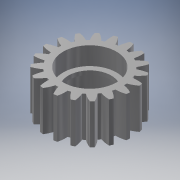
# Autodesk Inventor part: planet2_2
Saved by Autodesk Inventor 2019 (Build 230136000, 136)
## iProperties
Created: 2019-12-31
Part Number: planet2_2
Material: Steel
Document SubType Name: Modeling
Designer: louis
Categories: <?xml version="1.0" encoding="UTF-16"?> <MemberInstance><Categories><FamilyTemplate><FamilyTemplateParameter ValueType="xs:double" Id="1" ObjectReferenceKey="da_z" ObjectType="kUserParameterObject"/><FamilyTemplateParameter ValueType="xs:double" Id="2" ObjectReferenceKey="da_b" ObjectType="kUserParameterObject"/><FamilyTemplateParameter ValueType="xs:double" Id="3" ObjectReferenceKey="da_beta" ObjectType="kUserParameterObject"/><FamilyTemplateParameter ValueType="xs:double" Id="4" ObjectReferenceKey="da_da" ObjectType="kUserParameterObject"/><FamilyTemplateParameter ValueType="xs:double" Id="5" ObjectReferenceKey="da_aw" ObjectType="kUserParameterObject"/><FamilyTemplateParameter ValueType="xs:string" Id="6" ObjectReferenceKey="EAIAABAAAACIAQAAAAAAAIAAAAAAAAAA" ObjectType="83910656" SubObjectId="SurfaceGeometry"/></FamilyTemplate><ParamToTemplateMap><ParamToTemplate CategoryParameter="//CategoryParameter[@InternalName='046C89C9-8512-4d59-83FE-43B91F4F132A']" TemplateParameter="1"/><ParamToTemplate CategoryParameter="//CategoryParameter[@InternalName='2552DF32-E462-4b46-AEBF-C6C7768E72AC']" TemplateParameter="2"/><ParamToTemplate CategoryParameter="//CategoryParameter[@InternalName='C9EE641D-15FC-4fae-A226-E94C4372FDD7']" TemplateParameter="3"/><ParamToTemplate><ParamToTemplate CategoryParameter="//CategoryParameter[@InternalName='00B6519A-459B-49c7-AD84-2E56D39A5744']" ConstantValue="0.000000"/></ParamToTemplate><ParamToTemplate><ParamToTemplate CategoryParameter="//CategoryParameter[@InternalName='04B31F0E-C7A6-4894-AA32-9629BEFACF47']" ConstantValue="1.000000"/></ParamToTemplate><ParamToTemplate><ParamToTemplate CategoryParameter="//CategoryParameter[@InternalName='43CBEC2E-7847-49e7-A936-2F7889FCB2D9']" ConstantValue="0.250000"/></ParamToTemplate><ParamToTemplate><ParamToTemplate CategoryParameter="//CategoryParameter[@InternalName='B1EFC894-105D-4ebd-86BF-FA20ED196853']" ConstantValue="0.350000"/></ParamToTemplate><ParamToTemplate><ParamToTemplate CategoryParameter="//CategoryParameter[@InternalName='51175063-3D10-4879-93E8-6246FE8B403D']" ConstantValue="2060000000.000000"/></ParamToTemplate><ParamToTemplate><ParamToTemplate CategoryParameter="//CategoryParameter[@InternalName='A3A52E27-4454-46a9-B0BD-C932399B70AF']" ConstantValue="0.300000"/></ParamToTemplate><ParamToTemplate><ParamToTemplate CategoryParameter="//CategoryParameter[@InternalName='91B76062-C214-41d9-B1B9-14D2AB99603D']" ConstantValue="0.150000"/></ParamToTemplate><ParamToTemplate><ParamToTemplate CategoryParameter="//CategoryParameter[@InternalName='374E806E-8B8A-4dda-A9AA-1039D6500AD2']" ConstantValue="6.666667"/></ParamToTemplate><ParamToTemplate><ParamToTemplate CategoryParameter="//CategoryParameter[@InternalName='2D373A89-B862-43d6-8D0B-0CBF12AB9F6C']" ConstantValue="0.349066"/></ParamToTemplate><ParamToTemplate CategoryParameter="//CategoryParameter[@InternalName='37777632-D6A2-4fac-9D53-DB8ACD95C989']" TemplateParameter="4"/><ParamToTemplate CategoryParameter="//CategoryParameter[@InternalName='FD1017F1-B727-4f7e-9707-0F86F1FF9423']" TemplateParameter="5"/><ParamToTemplate><ParamToTemplate CategoryParameter="//CategoryParameter[@InternalName='9E1B4470-B2D3-4ff1-B813-535BB4CDF51A']" ConstantValue="3520000.000000"/></ParamToTemplate><ParamToTemplate><ParamToTemplate CategoryParameter="//CategoryParameter[@InternalName='F8452263-BFF6-458c-9FB1-07C4B99E95CD']" ConstantValue="11400000.000000"/></ParamToTemplate><ParamToTemplate><ParamToTemplate CategoryParameter="//CategoryParameter[@InternalName='3E3BB259-FD49-497f-8171-6EBC954A3479']" ConstantValue="2.000000"/></ParamToTemplate><ParamToTemplate CategoryParameter="//CategoryParameter[@InternalName='27C3BAF2-7550-4e4b-AE2C-0DB134B7D9B7']" TemplateParameter="6"/></ParamToTemplateMap><Category DisplayName="Gear" InternalName="DC85795E-93AB-48d5-8EEE-5A27447B64BD" Mnemonic="Gear"><CategoryParameter DisplayName="z" InternalName="046C89C9-8512-4d59-83FE-43B91F4F132A" Mnemonic="z"/><CategoryParameter DisplayName="b" InternalName="2552DF32-E462-4b46-AEBF-C6C7768E72AC" Mnemonic="b"/><CategoryParameter DisplayName="||b|" InternalName="C9EE641D-15FC-4fae-A226-E94C4372FDD7" Mnemonic="beta"/><CategoryParameter DisplayName="x" InternalName="00B6519A-459B-49c7-AD84-2E56D39A5744" Mnemonic="x"/><CategoryParameter DisplayName="a*" InternalName="04B31F0E-C7A6-4894-AA32-9629BEFACF47" Mnemonic="a"/><CategoryParameter DisplayName="c*" InternalName="43CBEC2E-7847-49e7-A936-2F7889FCB2D9" Mnemonic="c"/><CategoryParameter DisplayName="r|.f|*" InternalName="B1EFC894-105D-4ebd-86BF-FA20ED196853" Mnemonic="rf"/><CategoryParameter DisplayName="E" InternalName="51175063-3D10-4879-93E8-6246FE8B403D" Mnemonic="E"/><CategoryParameter DisplayName="||m|" InternalName="A3A52E27-4454-46a9-B0BD-C932399B70AF" Mnemonic="mi"/><Category DisplayName="SpurGear" InternalName="26C5A22E-A91E-4dfd-A3B3-23CCAFAE1764" Mnemonic="SpurGear"><CategoryParameter DisplayName="m" InternalName="91B76062-C214-41d9-B1B9-14D2AB99603D" Mnemonic="m"/><CategoryParameter DisplayName="P" InternalName="374E806E-8B8A-4dda-A9AA-1039D6500AD2" Mnemonic="PP"/><CategoryParameter DisplayName="||a|" InternalName="2D373A89-B862-43d6-8D0B-0CBF12AB9F6C" Mnemonic="alpha"/><CategoryParameter DisplayName="d|.a|" InternalName="37777632-D6A2-4fac-9D53-DB8ACD95C989" Mnemonic="da"/><CategoryParameter DisplayName="a|.w|" InternalName="FD1017F1-B727-4f7e-9707-0F86F1FF9423" Mnemonic="aw"/><CategoryParameter DisplayName="||s||.Flim|" InternalName="9E1B4470-B2D3-4ff1-B813-535BB4CDF51A" Mnemonic="sFlim"/><CategoryParameter DisplayName="||s||.Hlim|" InternalName="F8452263-BFF6-458c-9FB1-07C4B99E95CD" Mnemonic="sHlim"/><CategoryParameter DisplayName="類型" InternalName="3E3BB259-FD49-497f-8171-6EBC954A3479" Mnemonic="type"/><CategoryParameter DisplayName="PitchDiameter" InternalName="27C3BAF2-7550-4e4b-AE2C-0DB134B7D9B7" Mnemonic="IDS_PITCHDIAM"/></Category></Category></Categories></MemberInstance>
Density: 1 g/cm^3
Appearance: Steel
CustomPartVersion: 1
Author: louis
Autodesk Inventor part; units mm, degrees
sketch "Sketch1" plane through (0, 0, 0) normal (0, 0, 1) x (1, 0, 0)
  circle A0 centre (0, 0) radius 15.75
  dimension "d0" = 31.5
  constraints: 1 centre point
  measures "d0" diameter of A0
extrude "Extrusion1" add sketch "Sketch1" along normal blind 15
ref_plane "Work Plane2" through (0, 0, 7.5) normal (0, 0, 1) x (1, 0, 0)
sketch "Sketch2" plane through (0, 0, 0) normal (0, 0, -1) x (-1, 0, 0)
  circle A0 centre (0, 0) radius 15.75 projected
  circle A1 centre (0, 0) radius 14.25
  dimension "d3" = 28.5
  constraints: 1 centre point, 1 coincident
  measures "d3" diameter of A1
surface extrude "節圓直徑" sketch "Sketch2" against normal through all shown no curves A1
ref_plane "Work Plane8" through (0, 0, 0) normal (0.9863613, 0.1645946, 0) x (0, 0, 1)
ref_plane "Work Plane9" through (0, 0, 0) normal (1, 0, 0) x (0, 1, 0)
spur gear teeth "正齒輪" teeth 19 pitch diameter 28.5 tip diameter 31.5 root diameter 24.75 face width 15 start plane through (0, 0, 0) normal (0, 0, -1) x (-1, 0, 0)
sketch "草圖8" plane through (0, 0, 15) normal (0, 0, 1) x (1, 0, 0)
  circle A0 centre (0, 0) radius 10
  dimension "d73" = 20
  constraints: 1 centre point, 1 coincident
  measures "d73" diameter of A0
extrude "擠出7" cut sketch "草圖8" against normal blind 15
ref_plane "工作平面13" through (0, 0, 7.5) normal (0, 0, -1) x (-1, 0, 0)
sketch "草圖9" plane through (0, 0, 7.5) normal (0, 0, -1) x (-1, 0, 0)
  circle A0 centre (0, 0) radius 10 projected
  arc A1 (5.4351, 11.1176) -> (5.7253, 14.6726) centre (-6.3543, 13.8693) ccw projected
  arc A2 (6.3346, 10.6308) -> (5.4351, 11.1176) centre (0, 0) ccw projected
  arc A3 (9.152, 12.8181) -> (6.3346, 10.6308) centre (15.0864, 2.2662) ccw projected
  arc A4 (10.1792, 12.0186) -> (9.152, 12.8181) centre (0, 0) ccw projected
  arc A5 (8.7504, 8.7504) -> (10.1792, 12.0186) centre (-1.5066, 15.181) ccw projected
  arc A6 (9.4432, 7.998) -> (8.7504, 8.7504) centre (0, 0) ccw projected
  arc A7 (12.8181, 9.152) -> (9.4432, 7.998) centre (15.0048, -2.7551) ccw projected
  arc A8 (13.5301, 8.0622) -> (12.8181, 9.152) centre (0, 0) ccw projected
  arc A9 (11.1176, 5.4351) -> (13.5301, 8.0622) centre (3.5043, 14.8477) ccw projected
  arc A10 (11.5284, 4.4984) -> (11.1176, 5.4351) centre (0, 0) ccw projected
  arc A11 (15.0952, 4.494) -> (11.5284, 4.4984) centre (13.2972, -7.4779) ccw projected
  arc A12 (15.4148, 3.2321) -> (15.0952, 4.494) centre (0, 0) ccw projected
  arc A13 (12.28, 1.5307) -> (15.4148, 3.2321) centre (8.1354, 12.9054) ccw projected
  arc A14 (12.3644, 0.5114) -> (12.28, 1.5307) centre (0, 0) ccw projected
  arc A15 (15.7365, -0.6509) -> (12.3644, 0.5114) centre (10.1486, -11.3903) ccw projected
  arc A16 (15.629, -1.9482) -> (15.7365, -0.6509) centre (0, 0) ccw projected
  arc A17 (12.1116, -2.5395) -> (15.629, -1.9482) centre (11.885, 9.5645) ccw projected
  arc A18 (11.8605, -3.531) -> (12.1116, -2.5395) centre (0, 0) ccw projected
  arc A19 (14.6726, -5.7253) -> (11.8605, -3.531) centre (5.9003, -14.0684) ccw projected
  arc A20 (14.1497, -6.9173) -> (14.6726, -5.7253) centre (0, 0) ccw projected
  arc A21 (10.6308, -6.3346) -> (14.1497, -6.9173) centre (14.3466, 5.1873) ccw projected
  arc A22 (10.0714, -7.1908) -> (10.6308, -6.3346) centre (0, 0) ccw projected
  arc A23 (12.0186, -10.1792) -> (10.0714, -7.1908) centre (1.0126, -15.222) ccw projected
  arc A24 (11.1369, -11.1369) -> (12.0186, -10.1792) centre (0, 0) ccw projected
  arc A25 (7.998, -9.4432) -> (11.1369, -11.1369) centre (15.2536, 0.2479) ccw projected
  arc A26 (7.1908, -10.0714) -> (7.998, -9.4432) centre (0, 0) ccw projected
  arc A27 (8.0622, -13.5301) -> (7.1908, -10.0714) centre (-3.9848, -14.726) ccw projected
  arc A28 (6.9173, -14.1497) -> (8.0622, -13.5301) centre (0, 0) ccw projected
  arc A29 (4.4984, -11.5284) -> (6.9173, -14.1497) centre (14.5076, -4.7184) ccw projected
  arc A30 (3.531, -11.8605) -> (4.4984, -11.5284) centre (0, 0) ccw projected
  arc A31 (3.2321, -15.4148) -> (3.531, -11.8605) centre (-8.5504, -12.6342) ccw projected
  arc A32 (1.9482, -15.629) -> (3.2321, -15.4148) centre (0, 0) ccw projected
  arc A33 (0.5114, -12.3644) -> (1.9482, -15.629) centre (12.1895, -9.1734) ccw projected
  arc A34 (-0.5114, -12.3644) -> (0.5114, -12.3644) centre (0, 0) ccw projected
  arc A35 (-1.9482, -15.629) -> (-0.5114, -12.3644) centre (-12.1895, -9.1734) ccw projected
  arc A36 (-3.2321, -15.4148) -> (-1.9482, -15.629) centre (0, 0) ccw projected
  arc A37 (-3.531, -11.8605) -> (-3.2321, -15.4148) centre (8.5504, -12.6342) ccw projected
  arc A38 (-4.4984, -11.5284) -> (-3.531, -11.8605) centre (0, 0) ccw projected
  arc A39 (-6.9173, -14.1497) -> (-4.4984, -11.5284) centre (-14.5076, -4.7184) ccw projected
  arc A40 (-8.0622, -13.5301) -> (-6.9173, -14.1497) centre (0, 0) ccw projected
  arc A41 (-7.1908, -10.0714) -> (-8.0622, -13.5301) centre (3.9848, -14.726) ccw projected
  arc A42 (-7.998, -9.4432) -> (-7.1908, -10.0714) centre (0, 0) ccw projected
  arc A43 (-11.1369, -11.1369) -> (-7.998, -9.4432) centre (-15.2536, 0.2479) ccw projected
  arc A44 (-12.0186, -10.1792) -> (-11.1369, -11.1369) centre (0, 0) ccw projected
  arc A45 (-10.0714, -7.1908) -> (-12.0186, -10.1792) centre (-1.0126, -15.222) ccw projected
  arc A46 (-10.6308, -6.3346) -> (-10.0714, -7.1908) centre (0, 0) ccw projected
  arc A47 (-14.1497, -6.9173) -> (-10.6308, -6.3346) centre (-14.3466, 5.1873) ccw projected
  arc A48 (-14.6726, -5.7253) -> (-14.1497, -6.9173) centre (0, 0) ccw projected
  arc A49 (-11.8605, -3.531) -> (-14.6726, -5.7253) centre (-5.9003, -14.0684) ccw projected
  arc A50 (-12.1116, -2.5395) -> (-11.8605, -3.531) centre (0, 0) ccw projected
  arc A51 (-15.629, -1.9482) -> (-12.1116, -2.5395) centre (-11.885, 9.5645) ccw projected
  arc A52 (-15.7365, -0.6509) -> (-15.629, -1.9482) centre (0, 0) ccw projected
  arc A53 (-12.3644, 0.5114) -> (-15.7365, -0.6509) centre (-10.1486, -11.3903) ccw projected
  arc A54 (-12.28, 1.5307) -> (-12.3644, 0.5114) centre (0, 0) ccw projected
  arc A55 (-15.4148, 3.2321) -> (-12.28, 1.5307) centre (-8.1354, 12.9054) ccw projected
  arc A56 (-15.0952, 4.494) -> (-15.4148, 3.2321) centre (0, 0) ccw projected
  arc A57 (-11.5284, 4.4984) -> (-15.0952, 4.494) centre (-13.2972, -7.4779) ccw projected
  arc A58 (-11.1176, 5.4351) -> (-11.5284, 4.4984) centre (0, 0) ccw projected
  arc A59 (-13.5301, 8.0622) -> (-11.1176, 5.4351) centre (-3.5043, 14.8477) ccw projected
  arc A60 (-12.8181, 9.152) -> (-13.5301, 8.0622) centre (0, 0) ccw projected
  arc A61 (-9.4432, 7.998) -> (-12.8181, 9.152) centre (-15.0048, -2.7551) ccw projected
  arc A62 (-8.7504, 8.7504) -> (-9.4432, 7.998) centre (0, 0) ccw projected
  arc A63 (-10.1792, 12.0186) -> (-8.7504, 8.7504) centre (1.5066, 15.181) ccw projected
  arc A64 (-9.152, 12.8181) -> (-10.1792, 12.0186) centre (0, 0) ccw projected
  arc A65 (-6.3346, 10.6308) -> (-9.152, 12.8181) centre (-15.0864, 2.2662) ccw projected
  arc A66 (-5.4351, 11.1176) -> (-6.3346, 10.6308) centre (0, 0) ccw projected
  arc A67 (-5.7253, 14.6726) -> (-5.4351, 11.1176) centre (6.3543, 13.8693) ccw projected
  arc A68 (-4.494, 15.0952) -> (-5.7253, 14.6726) centre (0, 0) ccw projected
  arc A69 (-2.5395, 12.1116) -> (-4.494, 15.0952) centre (-13.5331, 7.0419) ccw projected
  arc A70 (-1.5307, 12.28) -> (-2.5395, 12.1116) centre (0, 0) ccw projected
  arc A71 (-0.6509, 15.7365) -> (-1.5307, 12.28) centre (10.5133, 11.0546) ccw projected
  arc A72 (0.6509, 15.7365) -> (-0.6509, 15.7365) centre (0, 0) ccw projected
  arc A73 (1.5307, 12.28) -> (0.6509, 15.7365) centre (-10.5133, 11.0546) ccw projected
  arc A74 (2.5395, 12.1116) -> (1.5307, 12.28) centre (0, 0) ccw projected
  arc A75 (4.494, 15.0952) -> (2.5395, 12.1116) centre (13.5331, 7.0419) ccw projected
  arc A76 (5.7253, 14.6726) -> (4.494, 15.0952) centre (0, 0) ccw projected
  circle A77 centre (0, 0) radius 8
  dimension "d77" = 2
  constraints: 1 centre point
  measures "d77" radial gap between concentric circles of A0 A77
extrude "擠出8" add sketch "草圖9" along normal mid plane 1.5 contours A0
equation "\"d0\" = da_da"
equation "\"d1\" = da_b"
equation "\"d3\" = da_dw"
equation "\"d16\" = da_aw"
equation "\"d43\" = da_aw"
equation "\"d46\" = da_aw"
equation "\"da_da\" = 31.5"
equation "\"da_b\" = 15"
equation "\"da_dw\" = 28.5"
equation "\"da_aw\" = 57"
body "Solid1"
body "Srf1"
